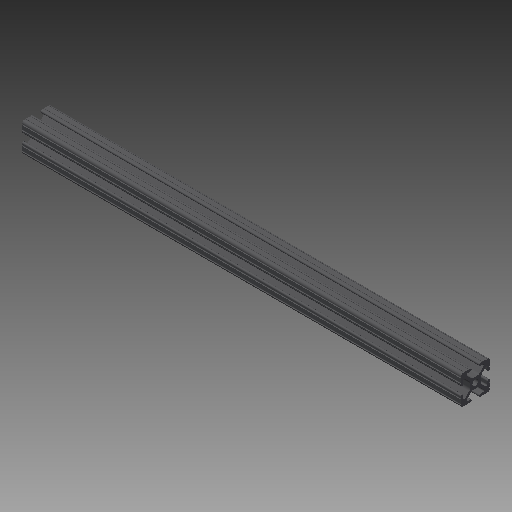
# Autodesk Inventor part: 1010-15-CL
Saved by Autodesk Inventor 2017 SP1 (Build 210196100, 196)
## iProperties
Category: PARTsolutions
Company: 8020
Created: 2016-04-02
Part Number: 1010-15-CL
Catalog Web Link: www.cadenas.de
Description: 1010-T-Slotted Profile - 10 Series
Vendor: 8020
Document SubType Name: Modeling
Designer: psAdmin
Manufacturer: 8020
Mass: 106.554 g
Surface Area: 856.785 cm^2
Volume: 106.554 cm^3
Density: 1 g/cm^3
Material: Generic
Appearance: PSOLRGB-175-175-175
PSOL_IDENT_0: {$CADENAS_DATA\23d-libs\8020\inch\profiles\10_series\1010.prj},161 {VTYP=3D},{NB=1010-15-CL},{LINA=1
PSOL_IDENT_1: 010-15},{NN=1010},{DATE=03.04.2014 11:10:31},{GEOMDATE=03.04.2014 11:10:00},{VERSION=},{LINEID=10},{
PSOL_IDENT_2: LINESUBID=-1},{WBVAR=LS,L}  {NB=1010-15-CL},{LINA=1010-15},{KT=DUMMY},{PN=1010-15},{SERIES=1010},{MA
PSOL_IDENT_3: T=6105-T5 Aluminum},{FIN=Clear Anodize},{LS=-CL},{L=15.000},{W=.5097},{LALG=[1:242/0.005]},{LPN= },{
PSOL_IDENT_4: MIX=.0442},{MIY=.0442},{EA=.4379}
NN: 1010
NT: T-Slotted Profile - 10 Series
NB: 1010-15-CL
NBSYN: $PN.$LS.
LINA: 1010-15
PN: 1010-15
SERIES: 1010
MAT: 6105-T5 Aluminum
FIN: Clear Anodize
LS: Custom Length
L: 15.000
W: .5097
MIX: .0442
MIY: .0442
EA: .4379
SUPPLIER: 8020
ARTICLENO: 1010-15-CL
BOMINFO: 1010-15
CREATOR: CADENAS GmbH
Title: 1010-15
Author: Cadenas PARTsolutions
Comments: T-Slotted Profile - 10 Series
Autodesk Inventor part; units mm, degrees
sketch "Sketch_1" plane through (0, 0, 0) normal (0, 0, 1) x (1, 0, 0)
  arc A0 (-12.6998, -10.5664) -> (-10.5664, -12.6998) centre (-10.5918, -10.5918) ccw
  arc A1 (-9.5504, -12.7) -> (-10.5664, -12.6998) centre (-10.0584, -12.7) ccw
  line L0 (-9.5504, -12.7) -> (-6.3331, -12.7)
  arc A2 (-5.3171, -12.7) -> (-6.3331, -12.7) centre (-5.8251, -12.7) ccw
  line L1 (-5.3171, -12.7) -> (-4.3434, -12.7)
  arc A3 (-4.3434, -12.7) -> (-4.3434, -10.4902) centre (-4.3434, -11.5951) ccw
  line L2 (-4.3434, -10.4902) -> (-6.4748, -10.4902)
  arc A4 (-7.1932, -8.7558) -> (-6.4748, -10.4902) centre (-6.4748, -9.4742) ccw
  line L3 (-7.1932, -8.7558) -> (-3.8632, -5.4257)
  arc A5 (-1.6181, -4.4958) -> (-3.8632, -5.4257) centre (-1.6181, -7.6708) ccw
  line L4 (-1.6181, -4.4958) -> (1.6181, -4.4958)
  arc A6 (3.8632, -5.4257) -> (1.6181, -4.4958) centre (1.6181, -7.6708) ccw
  line L5 (3.8632, -5.4257) -> (7.1932, -8.7558)
  arc A7 (6.4748, -10.4902) -> (7.1932, -8.7558) centre (6.4748, -9.4742) ccw
  line L6 (6.4748, -10.4902) -> (4.3434, -10.4902)
  arc A8 (4.3434, -10.4902) -> (4.3434, -12.7) centre (4.3434, -11.5951) ccw
  line L7 (4.3434, -12.7) -> (5.3171, -12.7)
  arc A9 (6.3331, -12.7) -> (5.3171, -12.7) centre (5.8251, -12.7) ccw
  line L8 (6.3331, -12.7) -> (9.5504, -12.7)
  arc A10 (10.5664, -12.6998) -> (9.5504, -12.7) centre (10.0584, -12.7) ccw
  arc A11 (10.5664, -12.6998) -> (12.6998, -10.5664) centre (10.5918, -10.5918) ccw
  arc A12 (12.7, -9.5504) -> (12.6998, -10.5664) centre (12.7, -10.0584) ccw
  line L9 (12.7, -9.5504) -> (12.7, -6.3331)
  arc A13 (12.7, -5.3171) -> (12.7, -6.3331) centre (12.7, -5.8251) ccw
  line L10 (12.7, -5.3171) -> (12.7, -4.3434)
  arc A14 (12.7, -4.3434) -> (10.4902, -4.3434) centre (11.5951, -4.3434) ccw
  line L11 (10.4902, -4.3434) -> (10.4902, -6.4748)
  arc A15 (8.7558, -7.1932) -> (10.4902, -6.4748) centre (9.4742, -6.4748) ccw
  line L12 (8.7558, -7.1932) -> (5.4257, -3.8632)
  arc A16 (4.4958, -1.6181) -> (5.4257, -3.8632) centre (7.6708, -1.6181) ccw
  line L13 (4.4958, -1.6181) -> (4.4958, 1.6181)
  arc A17 (5.4257, 3.8632) -> (4.4958, 1.6181) centre (7.6708, 1.6181) ccw
  line L14 (5.4257, 3.8632) -> (8.7558, 7.1932)
  arc A18 (10.4902, 6.4748) -> (8.7558, 7.1932) centre (9.4742, 6.4748) ccw
  line L15 (10.4902, 6.4748) -> (10.4902, 4.3434)
  arc A19 (10.4902, 4.3434) -> (12.7, 4.3434) centre (11.5951, 4.3434) ccw
  line L16 (12.7, 4.3434) -> (12.7, 5.3171)
  arc A20 (12.7, 6.3331) -> (12.7, 5.3171) centre (12.7, 5.8251) ccw
  line L17 (12.7, 6.3331) -> (12.7, 9.5504)
  arc A21 (12.6998, 10.5664) -> (12.7, 9.5504) centre (12.7, 10.0584) ccw
  arc A22 (12.6998, 10.5664) -> (10.5664, 12.6998) centre (10.5918, 10.5918) ccw
  arc A23 (9.5504, 12.7) -> (10.5664, 12.6998) centre (10.0584, 12.7) ccw
  line L18 (9.5504, 12.7) -> (6.3331, 12.7)
  arc A24 (5.3171, 12.7) -> (6.3331, 12.7) centre (5.8251, 12.7) ccw
  line L19 (5.3171, 12.7) -> (4.3434, 12.7)
  arc A25 (4.3434, 12.7) -> (4.3434, 10.4902) centre (4.3434, 11.5951) ccw
  line L20 (4.3434, 10.4902) -> (6.4748, 10.4902)
  arc A26 (7.1932, 8.7558) -> (6.4748, 10.4902) centre (6.4748, 9.4742) ccw
  line L21 (7.1932, 8.7558) -> (3.8632, 5.4257)
  arc A27 (1.6181, 4.4958) -> (3.8632, 5.4257) centre (1.6181, 7.6708) ccw
  line L22 (1.6181, 4.4958) -> (-1.6181, 4.4958)
  arc A28 (-3.8632, 5.4257) -> (-1.6181, 4.4958) centre (-1.6181, 7.6708) ccw
  line L23 (-3.8632, 5.4257) -> (-7.1932, 8.7558)
  arc A29 (-6.4748, 10.4902) -> (-7.1932, 8.7558) centre (-6.4748, 9.4742) ccw
  line L24 (-6.4748, 10.4902) -> (-4.3434, 10.4902)
  arc A30 (-4.3434, 10.4902) -> (-4.3434, 12.7) centre (-4.3434, 11.5951) ccw
  line L25 (-4.3434, 12.7) -> (-5.3171, 12.7)
  arc A31 (-6.3331, 12.7) -> (-5.3171, 12.7) centre (-5.8251, 12.7) ccw
  line L26 (-6.3331, 12.7) -> (-9.5504, 12.7)
  arc A32 (-10.5664, 12.6998) -> (-9.5504, 12.7) centre (-10.0584, 12.7) ccw
  arc A33 (-10.5664, 12.6998) -> (-12.6998, 10.5664) centre (-10.5918, 10.5918) ccw
  arc A34 (-12.7, 9.5504) -> (-12.6998, 10.5664) centre (-12.7, 10.0584) ccw
  line L27 (-12.7, 9.5504) -> (-12.7, 6.3331)
  arc A35 (-12.7, 5.3171) -> (-12.7, 6.3331) centre (-12.7, 5.8251) ccw
  line L28 (-12.7, 5.3171) -> (-12.7, 4.3434)
  arc A36 (-12.7, 4.3434) -> (-10.4902, 4.3434) centre (-11.5951, 4.3434) ccw
  line L29 (-10.4902, 4.3434) -> (-10.4902, 6.4748)
  arc A37 (-8.7558, 7.1932) -> (-10.4902, 6.4748) centre (-9.4742, 6.4748) ccw
  line L30 (-8.7558, 7.1932) -> (-5.4257, 3.8632)
  arc A38 (-4.4958, 1.6181) -> (-5.4257, 3.8632) centre (-7.6708, 1.6181) ccw
  line L31 (-4.4958, 1.6181) -> (-4.4958, -1.6181)
  arc A39 (-5.4257, -3.8632) -> (-4.4958, -1.6181) centre (-7.6708, -1.6181) ccw
  line L32 (-5.4257, -3.8632) -> (-8.7558, -7.1932)
  arc A40 (-10.4902, -6.4748) -> (-8.7558, -7.1932) centre (-9.4742, -6.4748) ccw
  line L33 (-10.4902, -6.4748) -> (-10.4902, -4.3434)
  arc A41 (-10.4902, -4.3434) -> (-12.7, -4.3434) centre (-11.5951, -4.3434) ccw
  line L34 (-12.7, -4.3434) -> (-12.7, -5.3171)
  arc A42 (-12.7, -6.3331) -> (-12.7, -5.3171) centre (-12.7, -5.8251) ccw
  line L35 (-12.7, -6.3331) -> (-12.7, -9.5504)
  arc A43 (-12.6998, -10.5664) -> (-12.7, -9.5504) centre (-12.7, -10.0584) ccw
  circle A44 centre (0, 0) radius 2.6035
  constraints: 88 point on circle, 72 end point, 45 centre point, 14 horizontal, 14 vertical, 179 other
extrude "Extrusion1" add sketch "Sketch_1" against normal blind 381
ref_plane "b1_XY" through (-12.7, 0, -190.5) normal (1, 0, 0) x (0, 0, -1)
ref_plane "b1_YZ" through (-12.7, 0, -190.5) normal (0, 0, -1) x (0, 1, 0)
ref_plane "b1_ZX" through (-12.7, 0, -190.5) normal (0, 1, 0) x (1, 0, 0)
ref_plane "b2_XY" through (12.7, 0, -190.5) normal (1, 0, 0) x (0, 0, -1)
ref_plane "b2_YZ" through (12.7, 0, -190.5) normal (0, 0, -1) x (0, 1, 0)
ref_plane "b2_ZX" through (12.7, 0, -190.5) normal (0, 1, 0) x (1, 0, 0)
ref_plane "profile1010_XY" through (0, 0, -190.5) normal (0, 0, 1) x (1, 0, 0)
ref_plane "profile1010_YZ" through (0, 0, -190.5) normal (1, 0, 0) x (0, 1, 0)
ref_plane "profile1010_ZX" through (0, 0, -190.5) normal (0, 1, 0) x (0, 0, 1)
sketch "Sketch4" plane through (12.7, 9.5504, 0) normal (1, 0, 0) x (0, 0, -1)
  line L0 (381, -3.2173) -> (381, 0) projected
  point P0 (0, -9.5504)
  point P1 (88.9, -9.5504)
  point P2 (63.5, -9.5504)
  point P3 (368.3, -9.5504)
  point P4 (12.7, -9.5504)
  point P5 (114.3, -9.5504)
  point P6 (139.7, -9.5504)
  point P7 (165.1, -9.5504)
  point P8 (215.9, -9.5504)
  point P9 (241.3, -9.5504)
  point P10 (266.7, -9.5504)
  point P11 (292.1, -9.5504)
  point P12 (317.5, -9.5504)
  dimension "d31" = 25.4
  dimension "d33" = 12.7
  dimension "d34" = 12.7
  dimension "d35" = 25.4
  dimension "d36" = 25.4
  dimension "d37" = 25.4
  dimension "d38" = 25.4
  dimension "d39" = 25.4
  dimension "d40" = 25.4
  dimension "d41" = 25.4
  dimension "d43" = 63.5
  dimension "d44" = 63.5
  constraints: 12 horizontal alignment
  measures "d31" distance of point (88.9, -9.55) point (63.5, -9.55)
  measures "d33" distance of point (0, -9.55) point (12.7, -9.55)
  measures "d34" distance from line of L0 point (368.3, -9.55)
  measures "d35" distance of point (114.3, -9.55) point (88.9, -9.55)
  measures "d36" distance of point (139.7, -9.55) point (114.3, -9.55)
  measures "d37" distance of point (165.1, -9.55) point (139.7, -9.55)
  measures "d38" distance of point (241.3, -9.55) point (215.9, -9.55)
  measures "d39" distance of point (266.7, -9.55) point (241.3, -9.55)
  measures "d40" distance of point (292.1, -9.55) point (266.7, -9.55)
  measures "d41" distance of point (317.5, -9.55) point (292.1, -9.55)
  measures "d43" distance from line of L0 point (317.5, -9.55)
  measures "d44" distance of point (63.5, -9.55) point (0, -9.55)
hole "Hole3" at (12.7, 0, -88.9) at (12.7, 0, -63.5) at (12.7, 0, -12.7) at (12.7, 0, -368.3) at (12.7, 0, -114.3) at (12.7, 0, -139.7) at (12.7, 0, -165.1) at (12.7, 0, -317.5) at (12.7, 0, -292.1) at (12.7, 0, -266.7) at (12.7, 0, -241.3) at (12.7, 0, -215.9) direction (-1, 0, 0) diameter 6.477 end through all
body "Solid1"
